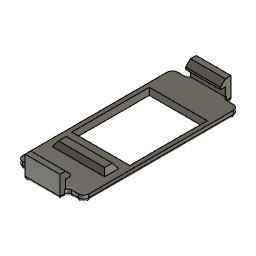
DHT22 lid (Autodesk Fusion 360 design; units mm, degrees)
Autodesk Fusion 360 part; units mm, degrees
note: some values were not read from the file. Chosen so that the rebuilt part matches the saved one: which face or edge a step refers to; which pieces of a blend or face edit are solid. Set by a fixed rule: which sketch regions a step uses.
sketch "base" plane through (0, 0, 0) normal (0, 0, 1) x (1, 0, 0)
  line L0 (19, 0) -> (19, 44.4)
  line L1 (0, 44.4) -> (0, 0)
  line L2 (14.5, 0) -> (14.5, -2.3)
  line L3 (14.5, -2.3) -> (4.5, -2.3)
  line L4 (4.5, -2.3) -> (4.5, 0)
  line L5 (14.5, 44.4) -> (14.5, 46.7)
  line L6 (14.5, 46.7) -> (4.5, 46.7)
  line L7 (4.5, 46.7) -> (4.5, 44.4)
  line L8 (19, 44.4) -> (14.5, 44.4)
  line L9 (4.5, 44.4) -> (0, 44.4)
  line L10 (0, 0) -> (4.5, 0)
  line L11 (14.5, 0) -> (19, 0)
  dimension "d1" = 19
  dimension "d2" = 44.4
  dimension "d60" = 10
  dimension "d61" = 2.3
  dimension "d62" = 4.5
  dimension "d63" = 10
  dimension "d64" = 2.3
  dimension "d65" = 4.5
  constraint horizontal L10
  constraint vertical L0
  constraint horizontal L8
  constraint vertical L1
  constraint coincident L1.end L10.start
  constraint vertical L2
  constraint horizontal L3
  constraint vertical L4
  constraint vertical L5
  constraint horizontal L6
  constraint vertical L7
  constraint coincident L7.end L8
  constraint collinear L8 L9
  constraint collinear L10 L11
  measures "d1" distance of L1.end L0.start
  measures "d2" distance of L1.end L1.start
  measures "d60" distance of L4.end L2.start
  measures "d61" distance of L4.end L3.end
  measures "d62" distance of L1.end L4
  measures "d63" distance of L7.end L5.start
  measures "d64" distance of L7.end L6.end
  measures "d65" distance of L1 L7
extrude "Extrude1" add sketch "base" along normal blind 2
fillet "Fillet3" radius 1 4 edges at (4.5, 0, 1) (14.5, 0, 1) (14.5, 44.4, 1) (4.5, 44.4, 1)
fillet "Fillet2" radius 1 1 faces at (7.5939, 29.6135, 0)
fillet "Fillet1" radius 1.5 8 edges at (19, 0, 1.5) (18.7071, 0.2929, 0.2929) (19, 44.4, 1.5) (18.7071, 44.1071, 0.2929) (0, 0, 1.5) (0, 44.4, 1.5) (0.2929, 0.2929, 0.2929) (0.2929, 44.1071, 0.2929)
sketch "holes" plane through (0, 0, 2) normal (0, 0, 1) x (-1, 0, 0)
  arc A0 (-19, -42.9) -> (-17.5, -44.4) centre (-17.5, -42.9) ccw
  line L0 (-17.5, -44.4) -> (-15.5, -44.4)
  arc A1 (-1.5, -44.4) -> (0, -42.9) centre (-1.5, -42.9) ccw
  line L1 (0, -42.9) -> (0, -1.5)
  arc A2 (0, -1.5) -> (-1.5, 0) centre (-1.5, -1.5) ccw
  line L2 (-1.5, 0) -> (-3.5, 0)
  arc A3 (-17.5, 0) -> (-19, -1.5) centre (-17.5, -1.5) ccw
  line L3 (-19, -1.5) -> (-19, -42.9)
  line L4 (-17.8, -36.6) -> (-17.8, -14.4)
  line L5 (-17.8, -14.4) -> (-1.2, -14.4)
  line L6 (-1.2, -14.4) -> (-1.2, -36.6)
  line L7 (-1.2, -36.6) -> (-17.8, -36.6)
  line L8 (-14.5, -45.4) -> (-14.5, -46.7)
  line L9 (-14.5, -46.7) -> (-4.5, -46.7)
  line L10 (-4.5, -46.7) -> (-4.5, -45.4)
  line L11 (-4.5, 1) -> (-4.5, 2.3)
  line L12 (-4.5, 2.3) -> (-14.5, 2.3)
  line L13 (-14.5, 2.3) -> (-14.5, 1)
  arc A4 (-14.5, -45.4) -> (-15.5, -44.4) centre (-15.5, -45.4) ccw
  arc A5 (-3.5, -44.4) -> (-4.5, -45.4) centre (-3.5, -45.4) ccw
  line L14 (-3.5, -44.4) -> (-1.5, -44.4)
  arc A6 (-4.5, 1) -> (-3.5, 0) centre (-3.5, 1) ccw
  arc A7 (-15.5, 0) -> (-14.5, 1) centre (-15.5, 1) ccw
  line L15 (-15.5, 0) -> (-17.5, 0)
  dimension "d15" = 14.4
  dimension "d16" = 1.2
  dimension "d17" = 16.6
  dimension "d57" = 22.2
  constraint vertical L4
  constraint horizontal L5
  constraint vertical L6
  measures "d15" distance of L2 L5
  measures "d16" distance of L3 L4
  measures "d17" distance of L6.end L4.start
  measures "d57" distance of L4.start L4.end
extrude "Extrude2" cut sketch "holes" against normal blind 2 contours L4 L5 L6 L7
sketch "pcb lock" plane through (0, 0, 2) normal (0, 0, 1) x (-1, 0, 0)
  line L0 (-17.8, -36.6) -> (-17.8, -14.4)
  line L1 (-17.8, -14.4) -> (-1.2, -14.4)
  line L2 (-1.2, -14.4) -> (-1.2, -36.6)
  arc A0 (-19, -42.9) -> (-17.5, -44.4) centre (-17.5, -42.9) ccw
  line L3 (-17.5, -44.4) -> (-15.5, -44.4)
  arc A1 (-1.5, -44.4) -> (0, -42.9) centre (-1.5, -42.9) ccw
  line L4 (0, -42.9) -> (0, -1.5)
  arc A2 (0, -1.5) -> (-1.5, 0) centre (-1.5, -1.5) ccw
  line L5 (-1.5, 0) -> (-3.5, 0)
  arc A3 (-17.5, 0) -> (-19, -1.5) centre (-17.5, -1.5) ccw
  line L6 (-19, -1.5) -> (-19, -42.9)
  line L7 (-2, -12) -> (-17, -12)
  line L8 (-17, -12) -> (-17, -8)
  line L9 (-17, -8) -> (-2, -8)
  line L10 (-2, -8) -> (-2, -12)
  line L11 (-1.2, -36.6) -> (-17.8, -36.6)
  line L12 (-14.5, -45.4) -> (-14.5, -46.7)
  line L13 (-14.5, -46.7) -> (-4.5, -46.7)
  line L14 (-4.5, -46.7) -> (-4.5, -45.4)
  line L15 (-4.5, 1) -> (-4.5, 2.3)
  line L16 (-4.5, 2.3) -> (-14.5, 2.3)
  line L17 (-14.5, 2.3) -> (-14.5, 1)
  arc A4 (-14.5, -45.4) -> (-15.5, -44.4) centre (-15.5, -45.4) ccw
  arc A5 (-3.5, -44.4) -> (-4.5, -45.4) centre (-3.5, -45.4) ccw
  line L18 (-3.5, -44.4) -> (-1.5, -44.4)
  arc A6 (-4.5, 1) -> (-3.5, 0) centre (-3.5, 1) ccw
  arc A7 (-15.5, 0) -> (-14.5, 1) centre (-15.5, 1) ccw
  line L19 (-15.5, 0) -> (-17.5, 0)
  dimension "d22" = 15
  dimension "d23" = 4
  dimension "d24" = 2
  dimension "d25" = 8
  constraint horizontal L7
  constraint vertical L8
  constraint horizontal L9
  constraint vertical L10
  measures "d22" distance of L7.start L7.end
  measures "d23" distance of L7.end L8.end
  measures "d24" distance of L4 L10
  measures "d25" distance of L5 L9
extrude "Extrude3" add sketch "pcb lock" along normal blind 1.4 contours L7 L8 L9 L10
chamfer "Chamfer1" distance 0.9 distance2 1.4 2 edges at (2, 10, 3.4) (9.5, 8, 3.4) 1 faces at (12, 10.6667, 3.4) measured on face at (12, 10.6667, 3.4) measured on face at (12, 10.6667, 3.4)
sketch "Sketch9" plane through (0, 0, 2) normal (0, 0, 1) x (-1, 0, 0)
  line L0 (-2, -8) -> (-2, -12)
  line L1 (-2, -12) -> (-17, -12)
  line L2 (-17, -12) -> (-17, -8)
  line L3 (-17, -8) -> (-2, -8)
  line L4 (-17.8, -14.4) -> (-1.2, -14.4)
  line L5 (-1.2, -14.4) -> (-1.2, -36.6)
  line L6 (-1.2, -36.6) -> (-17.8, -36.6)
  line L7 (-17.8, -36.6) -> (-17.8, -14.4)
  arc A0 (-19, -42.9) -> (-17.5, -44.4) centre (-17.5, -42.9) ccw
  line L8 (-17.5, -44.4) -> (-15.5, -44.4)
  arc A1 (-14.5, -45.4) -> (-15.5, -44.4) centre (-15.5, -45.4) ccw
  line L9 (-14.5, -45.4) -> (-14.5, -46.7)
  line L10 (-14.5, -46.7) -> (-4.5, -46.7)
  line L11 (-4.5, -46.7) -> (-4.5, -45.4)
  arc A2 (-3.5, -44.4) -> (-4.5, -45.4) centre (-3.5, -45.4) ccw
  line L12 (-3.5, -44.4) -> (-1.5, -44.4)
  arc A3 (-1.5, -44.4) -> (0, -42.9) centre (-1.5, -42.9) ccw
  line L13 (0, -42.9) -> (0, -1.5)
  arc A4 (0, -1.5) -> (-1.5, 0) centre (-1.5, -1.5) ccw
  line L14 (-1.5, 0) -> (-3.5, 0)
  arc A5 (-4.5, 1) -> (-3.5, 0) centre (-3.5, 1) ccw
  line L15 (-4.5, 1) -> (-4.5, 2.3)
  line L16 (-4.5, 2.3) -> (-14.5, 2.3)
  line L17 (-14.5, 2.3) -> (-14.5, 1)
  arc A6 (-15.5, 0) -> (-14.5, 1) centre (-15.5, 1) ccw
  line L18 (-15.5, 0) -> (-17.5, 0)
  arc A7 (-17.5, 0) -> (-19, -1.5) centre (-17.5, -1.5) ccw
  line L19 (-19, -1.5) -> (-19, -42.9)
  line L20 (-4.5, -46.7) -> (-14.5, -46.7)
  line L21 (-14.5, -46.7) -> (-14.5, -45.1)
  line L22 (-14.5, -45.1) -> (-4.5, -45.1)
  line L23 (-4.5, -45.1) -> (-4.5, -46.7)
  line L24 (-4.5, 2.3) -> (-14.5, 2.3)
  line L25 (-14.5, 2.3) -> (-14.5, 0.7)
  line L26 (-14.5, 0.7) -> (-4.5, 0.7)
  line L27 (-4.5, 0.7) -> (-4.5, 2.3)
  dimension "d68" = 10
  dimension "d69" = 1.6
  dimension "d70" = 10
  dimension "d71" = 1.6
  constraint horizontal L20
  constraint vertical L21
  constraint horizontal L22
  constraint vertical L23
  constraint coincident L10.end L11.start
  constraint horizontal L24
  constraint vertical L25
  constraint horizontal L26
  constraint vertical L27
  constraint coincident L15.end L16.start
  measures "d68" distance of L10.end L9.end
  measures "d69" distance of L10.end L22.end
  measures "d70" distance of L15.end L16.end
  measures "d71" distance of L15.end L26.end
extrude "Extrude9" add sketch "Sketch9" along normal blind 4.5 contours L9 L10 L11 L20 L21 L22 L23 | L15 L16 L17 L24 L25 L26 L27
sketch "Sketch10" plane through (0, -0.7, 0) normal (0, 1, 0) x (-1, 0, 0)
  line L0 (-14.5, 2) -> (-4.5, 2)
  line L1 (-4.5, 2) -> (-4.5, 6.5)
  line L2 (-4.5, 6.5) -> (-14.5, 6.5)
  line L3 (-14.5, 6.5) -> (-14.5, 2)
  line L4 (-14.5, 6.5) -> (-4.5, 6.5)
  line L5 (-4.5, 6.5) -> (-4.5, 4.5)
  line L6 (-4.5, 4.5) -> (-14.5, 4.5)
  line L7 (-14.5, 4.5) -> (-14.5, 6.5)
  dimension "d74" = 10
  dimension "d75" = 2
  constraint horizontal L4
  constraint vertical L5
  constraint horizontal L6
  constraint vertical L7
  constraint coincident L2.end L3.start
  measures "d74" distance of L2.end L1.end
  measures "d75" distance of L2.end L6.end
sketch "Sketch11" plane through (0, 45.1, 0) normal (0, -1, 0) x (1, 0, 0)
  line L0 (4.5, 2) -> (14.5, 2)
  line L1 (14.5, 2) -> (14.5, 6.5)
  line L2 (14.5, 6.5) -> (4.5, 6.5)
  line L3 (4.5, 6.5) -> (4.5, 2)
  line L4 (4.5, 6.5) -> (14.5, 6.5)
  line L5 (14.5, 6.5) -> (14.5, 4.5)
  line L6 (14.5, 4.5) -> (4.5, 4.5)
  line L7 (4.5, 4.5) -> (4.5, 6.5)
  dimension "d76" = 10
  dimension "d77" = 2
  constraint horizontal L4
  constraint vertical L5
  constraint horizontal L6
  constraint vertical L7
  constraint coincident L2.end L3.start
  measures "d76" distance of L2.end L1.end
  measures "d77" distance of L2.end L6.end
extrude "Extrude10" add sketch "Sketch11" along normal blind 1.4 contours L1 L2 L3 L4 L5 L6 L7
extrude "Extrude11" add sketch "Sketch10" along normal blind 1.4 contours L1 L2 L3 L4 L5 L6 L7
chamfer "Chamfer3" distance 1.4 angle 45 2 edges at (9.5, 43.7, 6.5) (9.5, 0.7, 6.5)
named bodies: "lid"
